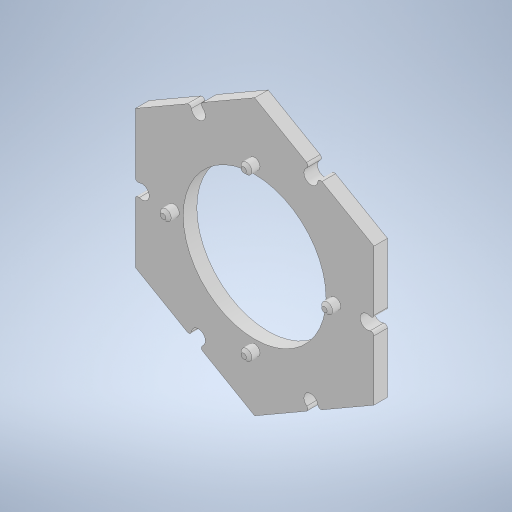
# Autodesk Inventor part: inner_top
Saved by Autodesk Inventor 2024 (Build 280153000, 153)
## iProperties
Created: 2024-03-18
Part Number: inner_top
Material: 일반
Document SubType Name: Modeling
Designer: SSAFY
Density: 1 g/cm^3
Appearance: 기본값
Author: SSAFY
Autodesk Inventor part; units mm, degrees
ref_plane "YZ Plane" through (0, 0, 0) normal (1, 0, 0) x (0, 1, 0)
ref_plane "XZ Plane" through (0, 0, 0) normal (0, 1, 0) x (-1, 0, 0)
ref_plane "XY Plane" through (0, 0, 0) normal (0, 0, 1) x (1, 0, 0)
sketch "스케치1" plane through (0, 0, 0) normal (0, 0, 1) x (1, 0, 0)
  line L0 (0, 45) -> (38.9711, 22.5)
  line L1 (38.9711, 22.5) -> (38.9711, -22.5)
  line L2 (38.9711, -22.5) -> (0, -45)
  line L3 (0, -45) -> (-38.9711, -22.5)
  line L4 (-38.9711, -22.5) -> (-38.9711, 22.5)
  line L5 (-38.9711, 22.5) -> (0, 45)
  line L6 (0, 50.7735) -> (43.9711, 25.3868)
  line L7 (43.9711, 25.3868) -> (43.9711, -25.3868)
  line L8 (43.9711, -25.3868) -> (0, -50.7735)
  line L9 (0, -50.7735) -> (-43.9711, -25.3868)
  line L10 (-43.9711, -25.3868) -> (-43.9711, 25.3868)
  line L11 (-43.9711, 25.3868) -> (0, 50.7735)
  circle A0 centre (-41.4711, 0) radius 2.5 construction
  circle A1 centre (-41.4711, 0) radius 2.6
  circle A2 centre (-20.7356, -35.9151) radius 2.6
  circle A3 centre (20.7356, -35.9151) radius 2.6
  circle A4 centre (41.4711, 0) radius 2.6
  circle A5 centre (20.7356, 35.9151) radius 2.6
  circle A6 centre (-20.7356, 35.9151) radius 2.6
  point P0 (0, 0)
  point P1 (0, 0)
  point P2 (-22.604, 37.7231)
  point P3 (-43.9711, 0.7141)
  point P4 (-43.9711, -0.7141)
  point P5 (-22.604, -37.7231)
  point P6 (-21.3671, -38.4372)
  point P7 (21.3671, -38.4372)
  point P8 (22.604, -37.7231)
  point P9 (43.9711, -0.7141)
  point P10 (43.9711, 0.7141)
  point P11 (22.604, 37.7231)
  point P12 (21.3671, 38.4372)
  point P13 (-21.3671, 38.4372)
  dimension "d0" = 45
  dimension "d1" = 5
  dimension "d2" = 5
  dimension "d3" = 5.2
  dimension "d6" = 360
  constraints: 24 end point, 7 centre point, 2 coincident, 1 tangent, 31 other
  measures "d0" distance of L3.end L4.end
  measures "d1" distance between parallel lines of L11 L5
  measures "d2" diameter of A0
  measures "d3" diameter of A1
extrude "돌출1" add sketch "스케치1" along normal blind 5 contours L5 A6 L11 L6 A5 L0 | L0 A5 L1 A4 L2 A3 L3 A2 L4 A1 L5 A6 | A5 L6 L7 A4 L1 L0 | L5 L4 A1 L10 L11 A6 | A4 L7 L8 A3 L2 L1 | L4 L3 A2 L9 L10 A1 | A3 L8 L9 A2 L3 L2
fillet "모깎기1" radius 1 12 edges at (-22.604, 37.7231, 2.5) (-21.3671, 38.4372, 2.5) (-43.9711, 0.7141, 2.5) (-43.9711, -0.7141, 2.5) (-22.604, -37.7231, 2.5) (-21.3671, -38.4372, 2.5) (21.3671, -38.4372, 2.5) (22.604, -37.7231, 2.5) (43.9711, -0.7141, 2.5) (43.9711, 0.7141, 2.5) (21.3671, 38.4372, 2.5) (22.604, 37.7231, 2.5)
sketch "스케치2" plane through (0, 0, 5) normal (0, 0, 1) x (1, 0, 0)
  circle A0 centre (0, 0) radius 26.325
  dimension "d11" = 52.65
  constraints: 1 centre point, 1 coincident
  measures "d11" diameter of A0
extrude "돌출2" cut sketch "스케치2" against normal through all
sketch "스케치3" plane through (0, 0, 5) normal (0, 0, 1) x (1, 0, 0)
  circle A0 centre (0, 0) radius 26.325 construction
  circle A1 centre (0, 0) radius 29.75
  circle A2 centre (0, 29.75) radius 2
  circle A3 centre (-29.75, 0) radius 2
  circle A4 centre (0, -29.75) radius 2
  circle A5 centre (29.75, 0) radius 2
  dimension "d14" = 59.5
  dimension "d15" = 4
  dimension "d18" = 360
  constraints: 4 centre point, 1 coincident, 1 vertical alignment, 11 other
  measures "d15" diameter of A2
extrude "돌출3" add sketch "스케치3" along normal blind 4 contours A1 A5 | A1 A5 | A2 A1 | A1 A2 | A4 A1 | A1 A4 | A3 A1 | A1 A3
chamfer "모따기1" distance 1 angle 45 4 edges at (-31.75, 0, 9) (-2, 29.75, 9) (27.75, 0, 9) (-2, -29.75, 9)
